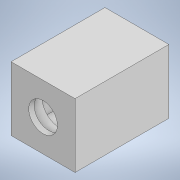
# Autodesk Inventor part: banebot soporte
Saved by Autodesk Inventor 2020.3 (Build 243373000, 373)
## iProperties
Created: 2021-01-22
Part Number: banebot soporte
Material: Generic
Document SubType Name: Modeling
Designer: Yu Jinyu
Density: 1 g/cm^3
Appearance: Default
Author: Yu Jinyu
Autodesk Inventor part; units mm, degrees
ref_plane "YZ Plane" through (0, 0, 0) normal (1, 0, 0) x (0, 1, 0)
ref_plane "XZ Plane" through (0, 0, 0) normal (0, 1, 0) x (-1, 0, 0)
ref_plane "XY Plane" through (0, 0, 0) normal (0, 0, 1) x (1, 0, 0)
sketch "Sketch1" plane through (0, 0, 0) normal (0, 0, 1) x (1, 0, 0)
  line L0 (-23.95, -23.95) -> (23.95, -23.95)
  line L1 (23.95, -23.95) -> (23.95, 23.95)
  line L2 (23.95, 23.95) -> (-23.95, 23.95)
  line L3 (-23.95, 23.95) -> (-23.95, -23.95)
  line L4 (-23.95, -23.95) -> (23.95, 23.95) construction
  line L5 (23.95, -23.95) -> (-23.95, 23.95) construction
  line L6 (28.95, 28.95) -> (28.95, -28.95)
  line L7 (28.95, -28.95) -> (-28.95, -28.95)
  line L8 (-28.95, -28.95) -> (-28.95, 28.95)
  line L9 (-28.95, 28.95) -> (28.95, 28.95)
  point P0 (0, 0)
  dimension "d0" = 47.9
  dimension "d1" = 47.9
  dimension "d2" = 5
  constraints: 20 end point, 4 parallel, 2 midpoint, 2 perpendicular, 1 horizontal, 3 other
  measures "d0" distance of L2.end L1.end
  measures "d1" distance between parallel lines of L0 L2
  measures "d2" distance between parallel lines of L1 L6
extrude "Extrusion1" add sketch "Sketch1" along normal blind 85
sketch "Sketch2" plane through (0, 0, 85) normal (0, 0, 1) x (1, 0, 0)
  line L0 (-23.95, 23.95) -> (23.95, 23.95) projected
  line L1 (-23.95, -23.95) -> (23.95, -23.95)
  line L2 (23.95, -23.95) -> (23.95, 23.95)
  line L3 (23.95, 23.95) -> (-23.95, 23.95)
  line L4 (-23.95, 23.95) -> (-23.95, -23.95)
  line L5 (-23.95, -23.95) -> (23.95, 23.95) construction
  line L6 (23.95, -23.95) -> (-23.95, 23.95) construction
  point P0 (0, 0)
  constraints: 12 end point, 2 midpoint, 2 parallel, 1 horizontal, 1 perpendicular
extrude "Extrusion2" add sketch "Sketch2" against normal blind 5
sketch "Sketch3" plane through (0, 0, 85) normal (0, 0, 1) x (1, 0, 0)
  circle A0 centre (0, 0) radius 16
  dimension "d7" = 32
  constraints: 1 centre point, 1 coincident
  measures "d7" diameter of A0
extrude "Extrusion3" cut sketch "Sketch3" along normal blind 8
sketch "Sketch4" plane through (-28.95, -28.95, 0) normal (-1, 0, 0) x (0, 0, 1)
  point P0 (0, 28.95)
sketch "Sketch5" plane through (0, 0, 80) normal (0, 0, -1) x (-1, 0, 0)
  line L0 (23.95, 23.95) -> (-23.95, 23.95) projected
  line L1 (-23.95, 23.95) -> (23.95, 23.95)
  line L2 (23.95, 23.95) -> (23.95, -23.9872)
  line L3 (23.95, -23.9872) -> (-23.95, -23.9872)
  line L4 (-23.95, -23.9872) -> (-23.95, 23.95)
  point P0 (0, 0)
  constraints: 8 end point, 2 parallel, 1 horizontal, 1 perpendicular
extrude "Extrusion4" add sketch "Sketch5" along normal blind 10
sketch "Sketch6" plane through (0, 0, 70) normal (0, 0, -1) x (-1, 0, 0)
  point P0 (0, 0)
sketch "Sketch7" plane through (0, 0, 70) normal (0, 0, -1) x (-1, 0, 0)
  circle A0 centre (0, 0) radius 16
  dimension "d12" = 32
  constraints: 1 centre point, 1 coincident
  measures "d12" diameter of A0
extrude "Extrusion5" cut sketch "Sketch7" against normal blind 10
sketch "Sketch8" plane through (0, 0, 85) normal (0, 0, 1) x (1, 0, 0)
  circle A0 centre (0, 0) radius 13
  dimension "d15" = 26
  constraints: 1 centre point, 1 coincident
  measures "d15" diameter of A0
extrude "Extrusion6" cut sketch "Sketch8" against normal blind 5
body "Solid1"
